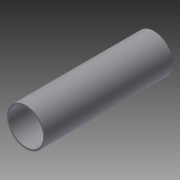
# Autodesk Inventor part: tubo_coprisiringa
Saved by Autodesk Inventor 2014 SP1 (Build 180222100, 222)
## iProperties
Created: 2015-04-15
Part Number: tubo_coprisiringa
Material: Generic
Document SubType Name: Modeling
Designer: Giorgio Nuzzo
Density: 1 g/cm^3
Appearance: Default
Author: Giorgio Nuzzo
Autodesk Inventor part; units mm, degrees
ref_plane "YZ Plane" through (0, 0, 0) normal (1, 0, 0) x (0, 1, 0)
ref_plane "XZ Plane" through (0, 0, 0) normal (0, 1, 0) x (-1, 0, 0)
ref_plane "XY Plane" through (0, 0, 0) normal (0, 0, 1) x (1, 0, 0)
sketch "Sketch1" plane through (0, 0, 0) normal (0, 1, 0) x (-1, 0, 0)
  circle A0 centre (0, 0) radius 17
  dimension "d0" = 34
  constraints: 1 centre point, 1 coincident
  measures "d0" diameter of A0
extrude "Extrusion1" add sketch "Sketch1" along normal blind 115
shell "Shell1" thickness 1.5 removed faces 2 at (6.0401, 0, -5.7878) at (6.0401, 115, -5.7878)
body "Solid1"
